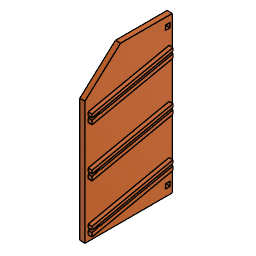
side-panel-left (Autodesk Fusion 360 design; units mm, degrees)
part number: 2026-08-18-20-10-10-569
Autodesk Fusion 360 part; units mm, degrees
sketch "Sketch1" plane through (0, 0, 0) normal (1, 0, 0) x (0, 0, -1)
  line L0 (0, 15) -> (0, 150)
  line L1 (0, 150) -> (-240, 150)
  line L2 (-240, 150) -> (-240, 70)
  line L3 (-240, 70) -> (-190, 15)
  line L4 (-190, 15) -> (0, 15)
extrude "Extrude1" add sketch "Sketch1" along normal blind 8 makes body 1
sketch "Sketch2" plane through (0, 0, 0) normal (1, 0, 0) x (0, 0, -1)
  line L0 (-9, 20) -> (-35.5696, 145)
  line L1 (-35.5696, 145) -> (-41.5696, 145)
  line L2 (-41.5696, 145) -> (-15, 20)
  line L3 (-15, 20) -> (-9, 20)
extrude "Extrude2" add sketch "Sketch2" along normal blind 6 from surface at 8 separate body makes body 2
sketch "Sketch3" plane through (0, 0, 0) normal (1, 0, 0) x (0, 0, -1)
  line L0 (-18.2, 20) -> (-44.7696, 145)
  line L1 (-44.7696, 145) -> (-49.7696, 145)
  line L2 (-49.7696, 145) -> (-23.2, 20)
  line L3 (-23.2, 20) -> (-18.2, 20)
extrude "Extrude3" add sketch "Sketch3" along normal blind 6 from surface at 8 separate body makes body 3
sketch "Sketch4" plane through (0, 0, 0) normal (1, 0, 0) x (0, 0, -1)
  line L0 (-16.2753, 26) -> (-17.2753, 28)
  line L1 (-17.2753, 28) -> (-18.3381, 31)
  line L2 (-18.3381, 31) -> (-17.7632, 33)
  line L3 (-17.7632, 33) -> (-16.2753, 26)
extrude "Extrude4" add sketch "Sketch4" along normal blind 6 from surface at 8 separate body makes body 4
sketch "Sketch5" plane through (0, 0, 0) normal (1, 0, 0) x (0, 0, -1)
  line L0 (-84, 20) -> (-110.5696, 145)
  line L1 (-110.5696, 145) -> (-116.5696, 145)
  line L2 (-116.5696, 145) -> (-90, 20)
  line L3 (-90, 20) -> (-84, 20)
extrude "Extrude5" add sketch "Sketch5" along normal blind 6 from surface at 8 separate body makes body 5
sketch "Sketch6" plane through (0, 0, 0) normal (1, 0, 0) x (0, 0, -1)
  line L0 (-93.2, 20) -> (-119.7696, 145)
  line L1 (-119.7696, 145) -> (-124.7696, 145)
  line L2 (-124.7696, 145) -> (-98.2, 20)
  line L3 (-98.2, 20) -> (-93.2, 20)
extrude "Extrude6" add sketch "Sketch6" along normal blind 6 from surface at 8 separate body makes body 6
sketch "Sketch7" plane through (0, 0, 0) normal (1, 0, 0) x (0, 0, -1)
  line L0 (-91.2753, 26) -> (-92.2753, 28)
  line L1 (-92.2753, 28) -> (-93.3381, 31)
  line L2 (-93.3381, 31) -> (-92.7632, 33)
  line L3 (-92.7632, 33) -> (-91.2753, 26)
extrude "Extrude7" add sketch "Sketch7" along normal blind 6 from surface at 8 separate body makes body 7
sketch "Sketch8" plane through (0, 0, 0) normal (1, 0, 0) x (0, 0, -1)
  line L0 (-159, 20) -> (-185.5696, 145)
  line L1 (-185.5696, 145) -> (-191.5696, 145)
  line L2 (-191.5696, 145) -> (-165, 20)
  line L3 (-165, 20) -> (-159, 20)
extrude "Extrude8" add sketch "Sketch8" along normal blind 6 from surface at 8 separate body makes body 8
sketch "Sketch9" plane through (0, 0, 0) normal (1, 0, 0) x (0, 0, -1)
  line L0 (-168.2, 20) -> (-194.7696, 145)
  line L1 (-194.7696, 145) -> (-199.7696, 145)
  line L2 (-199.7696, 145) -> (-173.2, 20)
  line L3 (-173.2, 20) -> (-168.2, 20)
extrude "Extrude9" add sketch "Sketch9" along normal blind 6 from surface at 8 separate body makes body 9
sketch "Sketch10" plane through (0, 0, 0) normal (1, 0, 0) x (0, 0, -1)
  line L0 (-166.2753, 26) -> (-167.2753, 28)
  line L1 (-167.2753, 28) -> (-168.3381, 31)
  line L2 (-168.3381, 31) -> (-167.7632, 33)
  line L3 (-167.7632, 33) -> (-166.2753, 26)
extrude "Extrude10" add sketch "Sketch10" along normal blind 6 from surface at 8 separate body makes body 10
combine "Combine1" operation add target body 1 tool bodies 2 3 4 5 6 7 8 9 10
sketch "Sketch11" plane through (0, 0, 0) normal (1, 0, 0) x (0, 0, -1)
  line L0 (-10.5, 139.5) -> (-10.5, 146.5)
  line L1 (-10.5, 146.5) -> (-17.5, 146.5)
  line L2 (-17.5, 146.5) -> (-17.5, 139.5)
  line L3 (-17.5, 139.5) -> (-10.5, 139.5)
extrude "Extrude11" cut sketch "Sketch11" along normal blind 30 from surface at -2 bodies 1
sketch "Sketch12" plane through (0, 0, 0) normal (1, 0, 0) x (0, 0, -1)
  line L0 (-222.5, 139.5) -> (-222.5, 146.5)
  line L1 (-222.5, 146.5) -> (-229.5, 146.5)
  line L2 (-229.5, 146.5) -> (-229.5, 139.5)
  line L3 (-229.5, 139.5) -> (-222.5, 139.5)
extrude "Extrude12" cut sketch "Sketch12" along normal blind 30 from surface at -2 bodies 1
named bodies: "Тело"
